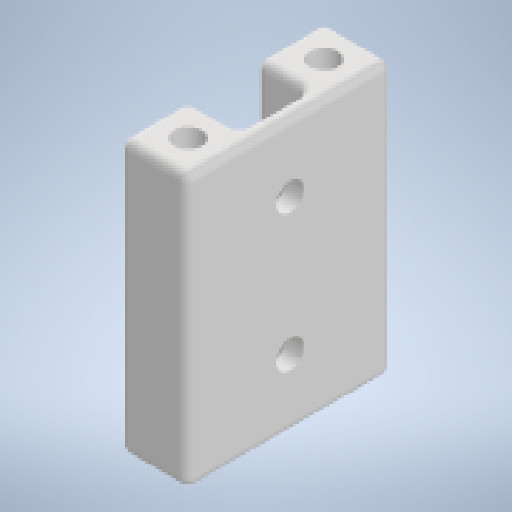
# Autodesk Inventor part: Connector plate
Saved by Autodesk Inventor 2023 (Build 270158000, 158)
## iProperties
Created: 2023-02-07
Part Number: Connector plate
Material: Generic
Document SubType Name: Modeling
Designer: Gabriel - T3 CAD
Density: 1 g/cm^3
Appearance: Default
Author: Gabriel - T3 CAD
Autodesk Inventor part; units mm, degrees
ref_plane "YZ Plane" through (0, 0, 0) normal (1, 0, 0) x (0, 1, 0)
ref_plane "XZ Plane" through (0, 0, 0) normal (0, 1, 0) x (-1, 0, 0)
ref_plane "XY Plane" through (0, 0, 0) normal (0, 0, 1) x (1, 0, 0)
sketch "Sketch1" plane through (0, 0, 0) normal (0, 1, 0) x (-1, 0, 0)
  line L0 (0, 0) -> (3.175, 0)
  line L1 (3.175, 0) -> (3.175, 38.1)
  line L2 (3.175, 38.1) -> (0, 38.1)
  line L3 (0, 38.1) -> (0, 0)
  circle A0 centre (6.35, 31.75) radius 2.5797
  circle A1 centre (6.35, 6.35) radius 2.5797
  line L4 (3.175, 38.1) -> (12.7, 38.1)
  line L5 (12.7, 38.1) -> (12.7, 0)
  line L6 (12.7, 0) -> (3.175, 0)
  line L7 (3.175, 0) -> (3.175, 38.1)
  line L8 (12.7, 25.4) -> (12.7, 12.7)
  line L9 (12.7, 12.7) -> (0, 12.7)
  line L10 (0, 12.7) -> (0, 25.4)
  line L11 (0, 25.4) -> (12.7, 25.4)
  point P0 (3.175, 12.7)
  point P1 (3.175, 25.4)
  dimension "d0" = 3.175
  dimension "d1" = 38.1
  dimension "d2" = 25.4
  dimension "d4" = 0
  dimension "d5" = 6.35
  dimension "d6" = 5.1594
  dimension "d7" = 5.1594
  dimension "d10" = 6.35
  dimension "d11" = 6.35
  dimension "d23" = 12.7
  dimension "d24" = 6.35
  constraints: 24 end point, 6 parallel, 4 point on line, 3 perpendicular, 2 centre point, 2 horizontal
  measures "d0" distance of L2.end L1.end
  measures "d1" distance of L1.end L0.end
  measures "d2" distance of A0.centre A1.centre
  measures "d4" horizontal distance of A1.centre A0.centre
  measures "d5" distance from line of A0.centre L2
  measures "d6" diameter of A0
  measures "d7" diameter of A1
  measures "d10" distance from line of A0.centre L11
  measures "d11" distance from line of A1.centre L9
  measures "d23" distance between parallel lines of L3 L5
  measures "d24" distance from line of L3 A0.centre
extrude "Extrusion1" add sketch "Sketch1" along normal blind 50.8 contours L3 L9 L1 L0 | L1 L9 L5 L6 | L3 L11 L1 L9 | L3 L2 L1 L11 | L1 L4 L5 L11
sketch "Sketch2" plane through (-3.175, 0, 12.7) normal (-1, 0, 0) x (0, 0, 1)
  circle A0 centre (6.35, 12.7) radius 2.5797
  circle A1 centre (6.35, 38.1) radius 2.5797
  line L0 (0, 0) -> (0, 50.8) projected
  line L1 (0, 0) -> (12.7, 0) projected
  point P0 (-12.7, 0)
  point P1 (6.35, 0)
  dimension "d14" = 0
  dimension "d15" = 25.4
  dimension "d16" = 5.1594
  dimension "d17" = 5.1594
  dimension "d18" = 6.35
  dimension "d19" = 12.7
  constraints: 2 centre point, 1 midpoint
  measures "d14" horizontal distance of A0.centre A1.centre
  measures "d15" distance of A0.centre A1.centre
  measures "d16" diameter of A1
  measures "d17" diameter of A0
  measures "d18" distance from line of L0 A0.centre
  measures "d19" distance of point (6.35, 0) A0.centre
extrude "Extrusion2" cut sketch "Sketch2" against normal blind 50.8
fillet "Fillet1" radius 1.5875 24 edges at (-3.175, 50.8, 19.05) (-7.9375, 50.8, 12.7) (-12.7, 50.8, 6.35) (-12.7, 50.8, 31.75) (0, 50.8, 19.05) (-3.175, 0, 19.05) (-3.175, 25.4, 12.7) (-3.175, 25.4, 25.4) (-12.7, 25.4, 12.7) (0, 25.4, 0) (0, 0, 19.05) (-12.7, 25.4, 0) (-12.7, 25.4, 25.4) (0, 25.4, 38.1) (-12.7, 25.4, 38.1) (-6.35, 50.8, 0) (-6.35, 50.8, 38.1) (-7.9375, 50.8, 25.4) (-12.7, 0, 6.35) (-7.9375, 0, 12.7) (-7.9375, 0, 25.4) (-6.35, 0, 38.1) (-12.7, 0, 31.75) (-6.35, 0, 0)
equation "\"d7\" = d6"
equation "\"d17\" = d16"
body "Solid1"
